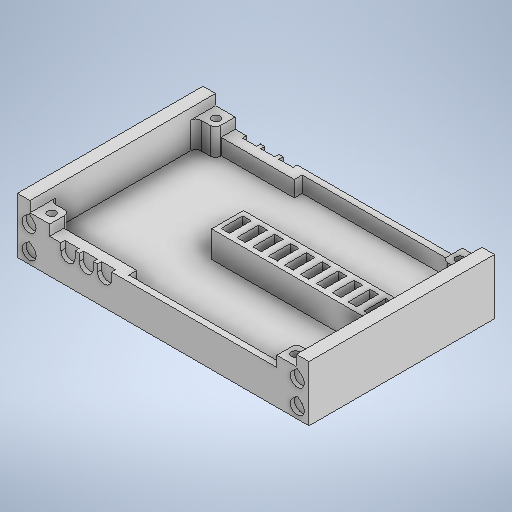
# Autodesk Inventor part: DisplayModuleHousing
Saved by Autodesk Inventor 2025.1 (Build 291241020, 241B)
## iProperties
Created: 2024-09-25
Part Number: DisplayModuleHousing
Material: Generic
Document SubType Name: Modeling
Designer: Si Teng Wu
Density: 1 g/cm^3
Appearance: Default
Author: Si Teng Wu
Autodesk Inventor part; units mm, degrees
ref_plane "YZ Plane" through (0, 0, 0) normal (1, 0, 0) x (0, 1, 0)
ref_plane "XZ Plane" through (0, 0, 0) normal (0, 1, 0) x (-1, 0, 0)
ref_plane "XY Plane" through (0, 0, 0) normal (0, 0, 1) x (1, 0, 0)
sketch "Sketch1" plane through (0, 0, 0) normal (0, 1, 0) x (-1, 0, 0)
  line L0 (55, 35) -> (-55, 35)
  line L1 (-55, 35) -> (-55, -35)
  line L2 (-55, -35) -> (55, -35)
  line L3 (55, -35) -> (55, 35)
  point P0 (0, 0)
  point P1 (-55, 0)
  point P2 (55, 0)
  dimension "d0" = 70
  dimension "d66" = 35
  dimension "d67" = 55
  dimension "d68" = 55
  constraints: 8 end point, 2 midpoint, 2 parallel, 1 horizontal, 1 perpendicular
  measures "d0" distance between parallel lines of L2 L0
  measures "d66" distance from line of L2 point (0, 0)
  measures "d67" distance of point (-55, 0) point (0, 0)
  measures "d68" distance of point (55, 0) point (0, 0)
extrude "Extrusion1" add sketch "Sketch1" along normal blind 21
sketch "Sketch2" plane through (0, 21, 0) normal (0, 1, 0) x (1, 0, 0)
  line L0 (-55, -35) -> (55, -35) projected
  line L1 (55, 35) -> (-55, 35) projected
  line L2 (50.25, -35) -> (-50.25, -35)
  line L3 (-50.25, -35) -> (-50.25, 35)
  line L4 (-50.25, 35) -> (50.25, 35)
  line L5 (50.25, 35) -> (50.25, -35)
  line L6 (-55, 35) -> (-55, -35) projected
  line L7 (55, -35) -> (55, 35) projected
  point P0 (0, 0)
  point P1 (-50.25, -35)
  dimension "d4" = 100.5
  dimension "d6" = 70
  dimension "d122" = 50.25
  constraints: 8 end point, 2 parallel, 2 point on line, 1 horizontal, 1 perpendicular
  measures "d4" distance between parallel lines of L3 L5
  measures "d6" distance between parallel lines of L1 L0
  measures "d122" distance from line of L3 point (0, 0)
extrude "Extrusion2" cut sketch "Sketch2" against normal blind 14 contours L3 L1 L5 L0
sketch "Sketch11" plane through (0, 7, 0) normal (0, 1, 0) x (1, 0, 0)
  line L0 (50.25, 35) -> (42.85, 35)
  line L1 (42.85, 35) -> (42.85, 27.5)
  line L2 (42.85, 27.5) -> (50.25, 27.5)
  line L3 (50.25, 27.5) -> (50.25, 35)
  circle A0 centre (46, 30.9) radius 1.55
  line L4 (50.25, 35) -> (50.25, -35) projected
  line L5 (50.25, -35) -> (42.85, -35)
  line L6 (42.85, -35) -> (42.85, -27.5)
  line L7 (42.85, -27.5) -> (50.25, -27.5)
  line L8 (50.25, -27.5) -> (50.25, -35)
  circle A1 centre (46, -31.1) radius 1.55
  line L9 (-42.85, 35) -> (-50.25, 35)
  line L10 (-50.25, 35) -> (-50.25, 27.5)
  line L11 (-50.25, 27.5) -> (-42.85, 27.5)
  line L12 (-42.85, 27.5) -> (-42.85, 35)
  circle A2 centre (-46, 30.9) radius 1.55
  line L13 (-50.25, 35) -> (50.25, 35) projected
  line L14 (-50.25, -35) -> (-50.25, 35) projected
  line L15 (-42.85, -35) -> (-50.25, -35)
  line L16 (-50.25, -35) -> (-50.25, -27.5)
  line L17 (-50.25, -27.5) -> (-42.85, -27.5)
  line L18 (-42.85, -27.5) -> (-42.85, -35)
  circle A3 centre (-46, -31.1) radius 1.55
  line L19 (50.25, -35) -> (-50.25, -35) projected
  point P0 (0, 0)
  point P1 (50.25, 31.25)
  point P2 (50.25, -8)
  point P3 (-42.85, 31.25)
  point P4 (-46.55, -35)
  point P5 (-50.25, -31.25)
  point P6 (50.25, -6)
  dimension "d89" = 7.5
  dimension "d91" = 3.1
  dimension "d92" = 4.25
  dimension "d93" = 7.4
  dimension "d334" = 3.9
  dimension "d335" = 7.5
  dimension "d336" = 7.4
  dimension "d338" = 92
  dimension "d339" = 62
  constraints: 32 end point, 8 parallel, 7 collinear, 4 centre point, 4 horizontal, 4 midpoint, 4 perpendicular, 3 equal radius, 2 horizontal alignment, 2 vertical alignment, 1 point on line
  measures "d89" distance between parallel lines of L17 L15
  measures "d91" diameter of A3
  measures "d92" distance from line of L16 A3.centre
  measures "d93" distance between parallel lines of L16 L18
  measures "d334" distance from line of L19 A3.centre
  measures "d335" distance between parallel lines of L11 L13
  measures "d336" distance between parallel lines of L6 L4
  measures "d338" distance of A0.centre A2.centre
  measures "d339" distance of A3.centre A2.centre
extrude "Extrusion10" add sketch "Sketch11" along normal blind 10 contours L3 L2 L1 L0 | L12 L11 L10 L9 | L4 L5 L6 L7 | L17 L18 L15 L14
fillet "Fillet5" radius 2 8 edges at (42.85, 12, 27.5) (50.25, 12, 27.5) (42.85, 12, -27.5) (50.25, 12, -27.5) (-42.85, 12, -27.5) (-50.25, 12, -27.5) (-50.25, 12, 27.5) (-42.85, 12, 27.5)
sketch "Sketch15" plane through (0, 7, 0) normal (0, 1, 0) x (1, 0, 0)
  circle A0 centre (46, -31.1) radius 1.55 projected
  circle A1 centre (46, -31.1) radius 1.6
  circle A2 centre (-46, -31.1) radius 1.55 projected
  circle A3 centre (-46, -31.1) radius 1.6
  circle A4 centre (-46, 30.9) radius 1.55 projected
  circle A5 centre (-46, 30.9) radius 1.6
  circle A6 centre (46, 30.9) radius 1.55 projected
  circle A7 centre (46, 30.9) radius 1.6
  point P0 (0, 0)
  constraints: 4 centre point, 4 coincident
extrude "Extrusion13" cut sketch "Sketch15" against normal through all contours A0 | A2 | A4 | A6
sketch "Sketch16" plane through (0, 0, 0) normal (0, -1, 0) x (1, 0, 0)
  line L0 (48.1, -28.2) -> (44.9, -28.2)
  line L1 (44.9, -28.2) -> (44.9, 28.2)
  line L2 (44.9, 28.2) -> (48.1, 28.2)
  line L3 (48.1, 28.2) -> (48.1, -28.2)
  line L4 (48.1, -28.2) -> (44.9, 28.2) construction
  line L5 (44.9, -28.2) -> (48.1, 28.2) construction
  line L6 (50.25, -25.5) -> (50.25, 25.5) projected
  line L7 (42.1, -28.2) -> (38.9, -28.2)
  line L8 (38.9, -28.2) -> (38.9, 28.2)
  line L9 (38.9, 28.2) -> (42.1, 28.2)
  line L10 (42.1, 28.2) -> (42.1, -28.2)
  line L11 (42.1, -28.2) -> (38.9, 28.2) construction
  line L12 (38.9, -28.2) -> (42.1, 28.2) construction
  line L13 (36.1, -28.2) -> (32.9, -28.2)
  line L14 (32.9, -28.2) -> (32.9, 28.2)
  line L15 (32.9, 28.2) -> (36.1, 28.2)
  line L16 (36.1, 28.2) -> (36.1, -28.2)
  line L17 (36.1, -28.2) -> (32.9, 28.2) construction
  line L18 (32.9, -28.2) -> (36.1, 28.2) construction
  line L19 (30.1, -28.2) -> (26.9, -28.2)
  line L20 (26.9, -28.2) -> (26.9, 28.2)
  line L21 (26.9, 28.2) -> (30.1, 28.2)
  line L22 (30.1, 28.2) -> (30.1, -28.2)
  line L23 (30.1, -28.2) -> (26.9, 28.2) construction
  line L24 (26.9, -28.2) -> (30.1, 28.2) construction
  line L25 (24.1, -28.2) -> (20.9, -28.2)
  line L26 (20.9, -28.2) -> (20.9, 28.2)
  line L27 (20.9, 28.2) -> (24.1, 28.2)
  line L28 (24.1, 28.2) -> (24.1, -28.2)
  line L29 (24.1, -28.2) -> (20.9, 28.2) construction
  line L30 (20.9, -28.2) -> (24.1, 28.2) construction
  line L31 (18.1, -28.2) -> (14.9, -28.2)
  line L32 (14.9, -28.2) -> (14.9, 28.2)
  line L33 (14.9, 28.2) -> (18.1, 28.2)
  line L34 (18.1, 28.2) -> (18.1, -28.2)
  line L35 (18.1, -28.2) -> (14.9, 28.2) construction
  line L36 (14.9, -28.2) -> (18.1, 28.2) construction
  line L37 (12.1, -28.2) -> (8.9, -28.2)
  line L38 (8.9, 28.2) -> (12.1, 28.2)
  line L39 (8.9, -28.2) -> (8.9, 28.2)
  line L40 (12.1, -28.2) -> (8.9, 28.2) construction
  line L41 (8.9, -28.2) -> (12.1, 28.2) construction
  line L42 (12.1, 28.2) -> (12.1, -28.2)
  line L43 (6.1, -28.2) -> (2.9, -28.2)
  line L44 (2.9, 28.2) -> (6.1, 28.2)
  line L45 (2.9, -28.2) -> (2.9, 28.2)
  line L46 (6.1, -28.2) -> (2.9, 28.2) construction
  line L47 (2.9, -28.2) -> (6.1, 28.2) construction
  line L48 (6.1, 28.2) -> (6.1, -28.2)
  line L49 (0.1, -28.2) -> (-3.1, -28.2)
  line L50 (-3.1, 28.2) -> (0.1, 28.2)
  line L51 (-3.1, -28.2) -> (-3.1, 28.2)
  line L52 (0.1, -28.2) -> (-3.1, 28.2) construction
  line L53 (-3.1, -28.2) -> (0.1, 28.2) construction
  line L54 (0.1, 28.2) -> (0.1, -28.2)
  line L55 (-5.9, -28.2) -> (-9.1, -28.2)
  line L56 (-9.1, 28.2) -> (-5.9, 28.2)
  line L57 (-9.1, -28.2) -> (-9.1, 28.2)
  line L58 (-5.9, -28.2) -> (-9.1, 28.2) construction
  line L59 (-9.1, -28.2) -> (-5.9, 28.2) construction
  line L60 (-5.9, 28.2) -> (-5.9, -28.2)
  line L61 (55, -35) -> (-55, -35) projected
  point P0 (46.5, 28.2)
  point P1 (40.5, 28.2)
  point P2 (34.5, 28.2)
  point P3 (28.5, 28.2)
  point P4 (22.5, 28.2)
  point P5 (16.5, 28.2)
  point P6 (10.5, 28.2)
  point P7 (4.5, 28.2)
  point P8 (-1.5, 28.2)
  point P9 (-7.5, 28.2)
  point P10 (46.5, -28.2)
  point P11 (40.5, 0)
  point P12 (46.5, 0)
  point P13 (34.5, 0)
  point P14 (40.5, 0)
  point P15 (28.5, 0)
  point P16 (34.5, 0)
  point P17 (22.5, 0)
  point P18 (28.5, 0)
  point P19 (16.5, 0)
  point P20 (22.5, 0)
  point P21 (10.5, 0)
  point P22 (16.5, 0)
  point P23 (4.5, 0)
  point P24 (10.5, 0)
  point P25 (-1.5, 0)
  point P26 (4.5, 0)
  point P27 (-7.5, 0)
  point P28 (-1.5, 0)
  point P29 (46.5, 0)
  dimension "d136" = 3.2
  dimension "d145" = 3.2
  dimension "d162" = 3.2
  dimension "d164" = 3.2
  dimension "d166" = 3.2
  dimension "d176" = 3.2
  dimension "d179" = 3.2
  dimension "d182" = 3.2
  dimension "d185" = 3.2
  dimension "d210" = 6
  dimension "d211" = 6
  dimension "d212" = 6
  dimension "d213" = 6
  dimension "d214" = 6
  dimension "d215" = 6
  dimension "d216" = 6
  dimension "d217" = 6
  dimension "d218" = 6
  dimension "d219" = 28.2
  dimension "d221" = 3.75
  dimension "d222" = 35
  constraints: 120 end point, 30 midpoint, 20 parallel, 19 collinear, 10 horizontal, 10 perpendicular
  measures "d136" distance between parallel lines of L1 L3
  measures "d145" distance between parallel lines of L14 L16
  measures "d162" distance between parallel lines of L20 L22
  measures "d164" distance between parallel lines of L26 L28
  measures "d166" distance between parallel lines of L32 L34
  measures "d176" distance between parallel lines of L39 L42
  measures "d179" distance between parallel lines of L45 L48
  measures "d182" distance between parallel lines of L51 L54
  measures "d185" distance between parallel lines of L57 L60
  measures "d210" distance of point (40.5, 0) point (46.5, 0)
  measures "d211" distance of point (34.5, 0) point (40.5, 0)
  measures "d212" distance of point (28.5, 0) point (34.5, 0)
  measures "d213" distance of point (22.5, 0) point (28.5, 0)
  measures "d214" distance of point (16.5, 0) point (22.5, 0)
  measures "d215" distance of point (10.5, 0) point (16.5, 0)
  measures "d216" distance of point (4.5, 0) point (10.5, 0)
  measures "d217" distance of point (-1.5, 0) point (4.5, 0)
  measures "d218" distance of point (-7.5, 0) point (-1.5, 0)
  measures "d219" distance from line of L0 point (46.5, 0)
  measures "d221" distance from line of L6 point (46.5, 0)
  measures "d222" distance from line of L61 point (46.5, 0)
extrude "Extrusion14" cut sketch "Sketch16" against normal blind 5
sketch "Sketch19" plane through (0, 7, 0) normal (0, 1, 0) x (1, 0, 0)
  line L0 (50.25, 35) -> (50.25, -35) projected
  line L1 (50.25, 6) -> (-10.75, 6)
  line L2 (-10.75, 6) -> (-10.75, -6)
  line L3 (-10.75, -6) -> (50.25, -6)
  line L4 (50.25, -6) -> (50.25, 6)
  line L5 (42.85, -35) -> (50.25, -35) projected
  point P0 (0, 0)
  dimension "d204" = 61
  dimension "d205" = 12
  dimension "d206" = 29
  constraints: 8 end point, 2 parallel, 1 horizontal, 1 perpendicular, 1 point on line
  measures "d204" distance between parallel lines of L2 L0
  measures "d205" distance between parallel lines of L3 L1
  measures "d206" distance between parallel lines of L5 L3
extrude "Extrusion16" add sketch "Sketch19" along normal up to surface (10 mm away)
sketch "Sketch17" plane through (0, 0, 0) normal (0, -1, 0) x (1, 0, 0)
  line L0 (48.1, 28.2) -> (48.1, -28.2) projected
  line L1 (44.9, 4.1) -> (48.1, 4.1)
  line L2 (48.1, 4.1) -> (48.1, -4.1)
  line L3 (48.1, -4.1) -> (44.9, -4.1)
  line L4 (44.9, -4.1) -> (44.9, 4.1)
  line L5 (44.9, 4.1) -> (48.1, -4.1) construction
  line L6 (48.1, 4.1) -> (44.9, -4.1) construction
  line L7 (44.9, -28.2) -> (44.9, 28.2) projected
  line L8 (42.1, 28.2) -> (42.1, -28.2) projected
  line L9 (38.9, 4.1) -> (42.1, 4.1)
  line L10 (42.1, 4.1) -> (42.1, -4.1)
  line L11 (42.1, -4.1) -> (38.9, -4.1)
  line L12 (38.9, -4.1) -> (38.9, 4.1)
  line L13 (38.9, 4.1) -> (42.1, -4.1) construction
  line L14 (42.1, 4.1) -> (38.9, -4.1) construction
  line L15 (36.1, 28.2) -> (36.1, -28.2) projected
  line L16 (32.9, 4.1) -> (36.1, 4.1)
  line L17 (36.1, 4.1) -> (36.1, -4.1)
  line L18 (36.1, -4.1) -> (32.9, -4.1)
  line L19 (32.9, -4.1) -> (32.9, 4.1)
  line L20 (32.9, 4.1) -> (36.1, -4.1) construction
  line L21 (36.1, 4.1) -> (32.9, -4.1) construction
  line L22 (30.1, 28.2) -> (30.1, -28.2) projected
  line L23 (26.9, 4.1) -> (30.1, 4.1)
  line L24 (30.1, 4.1) -> (30.1, -4.1)
  line L25 (30.1, -4.1) -> (26.9, -4.1)
  line L26 (26.9, -4.1) -> (26.9, 4.1)
  line L27 (26.9, 4.1) -> (30.1, -4.1) construction
  line L28 (30.1, 4.1) -> (26.9, -4.1) construction
  line L29 (24.1, 28.2) -> (24.1, -28.2) projected
  line L30 (20.9, 4.1) -> (24.1, 4.1)
  line L31 (24.1, 4.1) -> (24.1, -4.1)
  line L32 (24.1, -4.1) -> (20.9, -4.1)
  line L33 (20.9, -4.1) -> (20.9, 4.1)
  line L34 (20.9, 4.1) -> (24.1, -4.1) construction
  line L35 (24.1, 4.1) -> (20.9, -4.1) construction
  line L36 (18.1, 28.2) -> (18.1, -28.2) projected
  line L37 (14.9, 4.1) -> (18.1, 4.1)
  line L38 (18.1, 4.1) -> (18.1, -4.1)
  line L39 (18.1, -4.1) -> (14.9, -4.1)
  line L40 (14.9, -4.1) -> (14.9, 4.1)
  line L41 (14.9, 4.1) -> (18.1, -4.1) construction
  line L42 (18.1, 4.1) -> (14.9, -4.1) construction
  line L43 (12.1, 28.2) -> (12.1, -28.2) projected
  line L44 (8.9, 4.1) -> (12.1, 4.1)
  line L45 (12.1, 4.1) -> (12.1, -4.1)
  line L46 (12.1, -4.1) -> (8.9, -4.1)
  line L47 (8.9, -4.1) -> (8.9, 4.1)
  line L48 (8.9, 4.1) -> (12.1, -4.1) construction
  line L49 (12.1, 4.1) -> (8.9, -4.1) construction
  line L50 (2.9, 4.1) -> (6.1, 4.1)
  line L51 (6.1, 4.1) -> (6.1, -4.1)
  line L52 (6.1, -4.1) -> (2.9, -4.1)
  line L53 (2.9, -4.1) -> (2.9, 4.1)
  line L54 (2.9, 4.1) -> (6.1, -4.1) construction
  line L55 (6.1, 4.1) -> (2.9, -4.1) construction
  line L56 (-3.1, 4.1) -> (0.1, 4.1)
  line L57 (0.1, 4.1) -> (0.1, -4.1)
  line L58 (0.1, -4.1) -> (-3.1, -4.1)
  line L59 (-3.1, -4.1) -> (-3.1, 4.1)
  line L60 (-3.1, 4.1) -> (0.1, -4.1) construction
  line L61 (0.1, 4.1) -> (-3.1, -4.1) construction
  line L62 (-5.9, 28.2) -> (-5.9, -28.2) projected
  line L63 (-9.1, 4.1) -> (-5.9, 4.1)
  line L64 (-5.9, 4.1) -> (-5.9, -4.1)
  line L65 (-5.9, -4.1) -> (-9.1, -4.1)
  line L66 (-9.1, -4.1) -> (-9.1, 4.1)
  line L67 (-9.1, 4.1) -> (-5.9, -4.1) construction
  line L68 (-5.9, 4.1) -> (-9.1, -4.1) construction
  line L69 (38.9, -28.2) -> (38.9, 28.2) projected
  line L70 (32.9, -28.2) -> (32.9, 28.2) projected
  line L71 (26.9, -28.2) -> (26.9, 28.2) projected
  line L72 (20.9, -28.2) -> (20.9, 28.2) projected
  line L73 (14.9, -28.2) -> (14.9, 28.2) projected
  line L74 (8.9, -28.2) -> (8.9, 28.2) projected
  line L75 (2.9, -28.2) -> (2.9, 28.2) projected
  line L76 (-3.1, -28.2) -> (-3.1, 28.2) projected
  line L77 (0.1, 28.2) -> (0.1, -28.2) projected
  line L78 (6.1, 28.2) -> (6.1, -28.2) projected
  line L79 (12.1, 28.2) -> (12.1, -28.2) projected
  line L80 (-9.1, -28.2) -> (-9.1, 28.2) projected
  line L81 (55, -35) -> (-55, -35) projected
  point P0 (0, 0)
  point P1 (46.5, 0)
  point P2 (40.5, 0)
  point P3 (34.5, 0)
  point P4 (28.5, 0)
  point P5 (22.5, 0)
  point P6 (16.5, 0)
  point P7 (10.5, 0)
  point P8 (4.5, 0)
  point P9 (-1.5, 0)
  point P10 (-7.5, 0)
  point P11 (46.5, -4.1)
  point P12 (-5.9, 4.1)
  point P13 (12.1, 4.1)
  point P14 (24.1, 4.1)
  point P15 (42.1, 4.1)
  dimension "d200" = 4.1
  dimension "d201" = 35
  constraints: 120 end point, 23 collinear, 21 midpoint, 20 parallel, 16 point on line, 10 horizontal, 10 perpendicular
  measures "d200" distance of point (46.5, 0) point (46.5, -4.1)
  measures "d201" distance from line of L81 point (46.5, 0)
extrude "Extrusion15" cut sketch "Sketch17" against normal through all
chamfer "Chamfer3" distance 1 distance2 1.5 1 edges at (6.1, 5, -16.15) measured on face at (6.1, 1.6667, -20.1667)
chamfer "Chamfer4" distance 1 distance2 1.5 1 edges at (2.9, 5, -16.15) measured on face at (2.9, 1.6667, -12.1333)
chamfer "Chamfer5" distance 1 distance2 1.5 1 edges at (-3.1, 5, -16.15) measured on face at (-3.1, 1.6667, -12.1333)
chamfer "Chamfer6" distance 1 distance2 1.5 1 edges at (0.1, 5, -16.15) measured on face at (0.1, 1.6667, -20.1667)
chamfer "Chamfer7" distance 1 distance2 1.5 1 edges at (-5.9, 5, -16.15) measured on face at (-5.9, 1.6667, -20.1667)
chamfer "Chamfer8" distance 1 distance2 1.5 1 edges at (-9.1, 5, -16.15) measured on face at (-9.1, 1.6667, -12.1333)
chamfer "Chamfer9" distance 1 distance2 1.5 1 edges at (8.9, 5, -16.15) measured on face at (8.9, 1.6667, -12.1333)
chamfer "Chamfer10" distance 1 distance2 1.5 1 edges at (12.1, 5, -16.15) measured on face at (12.1, 1.6667, -20.1667)
chamfer "Chamfer11" distance 1 distance2 1.5 1 edges at (18.1, 5, -16.15) measured on face at (18.1, 1.6667, -20.1667)
chamfer "Chamfer12" distance 1 distance2 1.5 1 edges at (14.9, 5, -16.15) measured on face at (14.9, 3.3333, -20.1667)
chamfer "Chamfer13" distance 1 distance2 1.5 1 edges at (24.1, 5, -16.15) measured on face at (24.1, 1.6667, -20.1667)
chamfer "Chamfer14" distance 1 distance2 1.5 1 edges at (20.9, 5, -16.15) measured on face at (20.9, 1.6667, -12.1333)
chamfer "Chamfer15" distance 1 distance2 1.5 1 edges at (30.1, 5, -16.15) measured on face at (30.1, 1.6667, -20.1667)
chamfer "Chamfer16" distance 1 distance2 1.5 1 edges at (26.9, 5, -16.15) measured on face at (26.9, 1.6667, -12.1333)
chamfer "Chamfer17" distance 1 distance2 1.5 1 edges at (36.1, 5, -16.15) measured on face at (36.1, 1.6667, -20.1667)
chamfer "Chamfer18" distance 1 distance2 1.5 1 edges at (32.9, 5, -16.15) measured on face at (32.9, 1.6667, -12.1333)
chamfer "Chamfer19" distance 1 distance2 1.5 1 edges at (38.9, 5, -16.15) measured on face at (38.9, 1.6667, -12.1333)
chamfer "Chamfer20" distance 1 distance2 1.5 1 edges at (42.1, 5, -16.15) measured on face at (42.1, 1.6667, -20.1667)
chamfer "Chamfer21" distance 1.5 distance2 1 2 edges at (44.9, 5, -16.15) (48.1, 5, -16.15) measured on face at (45.9667, 5, -20.1667)
chamfer "Chamfer22" distance 1.5 distance2 1 2 edges at (44.9, 5, 16.15) (48.1, 5, 16.15) measured on face at (47.0333, 5, 12.1333)
chamfer "Chamfer23" distance 1.5 distance2 1 2 edges at (38.9, 5, 16.15) (42.1, 5, 16.15) measured on face at (39.9667, 5, 20.1667)
chamfer "Chamfer24" distance 1.5 distance2 1 2 edges at (32.9, 5, 16.15) (36.1, 5, 16.15) measured on face at (33.9667, 5, 20.1667)
chamfer "Chamfer25" distance 1.5 distance2 1 2 edges at (30.1, 5, 16.15) (26.9, 5, 16.15) measured on face at (27.9667, 5, 20.1667)
chamfer "Chamfer26" distance 1.5 distance2 1 2 edges at (20.9, 5, 16.15) (24.1, 5, 16.15) measured on face at (23.0333, 5, 12.1333)
chamfer "Chamfer27" distance 1.5 distance2 1 2 edges at (18.1, 5, 16.15) (14.9, 5, 16.15) measured on face at (15.9667, 5, 12.1333)
chamfer "Chamfer28" distance 1.5 distance2 1 2 edges at (8.9, 5, 16.15) (12.1, 5, 16.15) measured on face at (11.0333, 5, 12.1333)
chamfer "Chamfer29" distance 1.5 distance2 1 2 edges at (2.9, 5, 16.15) (6.1, 5, 16.15) measured on face at (5.0333, 5, 12.1333)
chamfer "Chamfer30" distance 1.5 distance2 1 2 edges at (-3.1, 5, 16.15) (0.1, 5, 16.15) measured on face at (-0.9667, 5, 12.1333)
chamfer "Chamfer31" distance 1.5 distance2 1 2 edges at (-5.9, 5, 16.15) (-9.1, 5, 16.15) measured on face at (-6.9667, 5, 12.1333)
sketch "Sketch20" plane through (0, 0, 0) normal (0, -1, 0) x (1, 0, 0)
  circle A0 centre (-46, -30.9) radius 1.55
  circle A1 centre (-46, -30.9) radius 1.55 projected
  circle A2 centre (-46, 31.1) radius 1.55
  circle A3 centre (46, 31.1) radius 1.55
  circle A4 centre (46, -30.9) radius 1.55
  circle A5 centre (-46, 31.1) radius 1.55 projected
  circle A6 centre (46, 31.1) radius 1.55 projected
  circle A7 centre (46, -30.9) radius 1.55 projected
  point P0 (0, 0)
  constraints: 4 centre point, 4 concentric, 4 equal radius
extrude "Extrusion17" add sketch "Sketch20" against normal blind 5
sketch "Sketch21" plane through (0, 7, 0) normal (0, 1, 0) x (1, 0, 0)
  line L0 (-42.85, -32.7) -> (42.85, -32.7)
  line L1 (42.85, -32.7) -> (42.85, -35)
  line L2 (42.85, -35) -> (-42.85, -35)
  line L3 (-42.85, -35) -> (-42.85, -32.7)
  line L4 (42.85, -35) -> (-42.85, -35) projected
  line L5 (-42.85, -35) -> (-42.85, -29.5) projected
  line L6 (42.85, -29.5) -> (42.85, -35) projected
  line L7 (-42.85, 35) -> (42.85, 35)
  line L8 (42.85, 35) -> (42.85, 32.7)
  line L9 (42.85, 32.7) -> (-42.85, 32.7)
  line L10 (-42.85, 32.7) -> (-42.85, 35)
  line L11 (-42.85, 29.5) -> (-42.85, 35) projected
  line L12 (-42.85, 35) -> (42.85, 35) projected
  line L13 (42.85, 35) -> (42.85, 29.5) projected
  line L14 (-42.85, -29.7) -> (-15.25, -29.7)
  line L15 (-15.25, -29.7) -> (-15.25, -32.7)
  line L16 (-15.25, -32.7) -> (-42.85, -32.7)
  line L17 (-42.85, -32.7) -> (-42.85, -29.7)
  line L18 (-42.85, 32.7) -> (-15.25, 32.7)
  line L19 (-15.25, 32.7) -> (-15.25, 29.7)
  line L20 (-15.25, 29.7) -> (-42.85, 29.7)
  line L21 (-42.85, 29.7) -> (-42.85, 32.7)
  line L22 (-50.25, -35) -> (-50.25, 35) projected
  point P0 (0, 0)
  point P1 (-15.25, 31.2)
  point P2 (-15.25, 32.7)
  dimension "d353" = 2.3
  dimension "d354" = 2.3
  dimension "d355" = 35
  dimension "d356" = 3
  dimension "d357" = 3
  constraints: 32 end point, 11 collinear, 8 parallel, 4 horizontal, 4 perpendicular, 1 midpoint
  measures "d353" distance between parallel lines of L0 L2
  measures "d354" distance between parallel lines of L9 L7
  measures "d355" distance from line of L22 point (-15.25, 31.2)
  measures "d356" distance between parallel lines of L18 L20
  measures "d357" distance between parallel lines of L0 L14
extrude "Extrusion18" add sketch "Sketch21" along normal blind 6
sketch "Sketch12" plane through (-42.85, 7, 35) normal (0, 0, 1) x (1, 0, 0)
  circle A0 centre (-7.75, 6) radius 2.65
  line L0 (-7.4, 10) -> (0, 10) projected
  line L1 (-12.15, -7) -> (-12.15, 14) projected
  circle A1 centre (93.45, 6) radius 2.65
  line L2 (97.85, -7) -> (97.85, 14) projected
  line L3 (85.7, 10) -> (93.1, 10) projected
  circle A2 centre (93.45, -3) radius 2.65
  circle A3 centre (-7.75, -3) radius 2.65
  line L4 (-9.4811, -0.9936) -> (-7.75, 0.5)
  line L5 (-7.75, 0.5) -> (-6.0189, -0.9936)
  line L6 (-9.4811, 8.0064) -> (-7.75, 9.5)
  line L7 (-7.75, 9.5) -> (-6.0189, 8.0064)
  line L8 (91.7189, -0.9936) -> (93.45, 0.5)
  line L9 (93.45, 0.5) -> (95.1811, -0.9936)
  line L10 (91.7189, 8.0064) -> (93.45, 9.5)
  line L11 (93.45, 9.5) -> (95.1811, 8.0064)
  line L12 (85.7, 0) -> (0, 0) projected
  line L13 (-12.15, -7) -> (97.85, -7) projected
  circle A4 centre (6.9, 3.35) radius 2.65
  circle A5 centre (13.8, 3.35) radius 2.65
  circle A6 centre (20.7, 3.35) radius 2.65
  line L14 (0, 6) -> (0, 0) projected
  line L15 (9.55, 3.35) -> (4.25, 3.35)
  line L16 (4.25, 3.35) -> (4.25, 6)
  line L17 (4.25, 6) -> (9.55, 6)
  line L18 (9.55, 6) -> (9.55, 3.35)
  line L19 (11.15, 3.35) -> (16.45, 3.35)
  line L20 (16.45, 3.35) -> (16.45, 6)
  line L21 (16.45, 6) -> (11.15, 6)
  line L22 (11.15, 6) -> (11.15, 3.35)
  line L23 (0, 6) -> (27.6, 6) projected
  line L24 (18.05, 3.35) -> (23.35, 3.35)
  line L25 (23.35, 3.35) -> (23.35, 6)
  line L26 (23.35, 6) -> (18.05, 6)
  line L27 (18.05, 6) -> (18.05, 3.35)
  line L28 (0, 6) -> (85.7, 6) projected
  point P0 (42.85, -7)
  point P1 (18.9615, 0)
  point P2 (22.4385, 0)
  point P3 (12.0615, 0)
  point P4 (15.5385, 0)
  point P5 (5.1615, 0)
  point P6 (8.6385, 0)
  point P7 (16.45, 3.35)
  point P8 (4.25, 3.35)
  point P9 (6.9, 3.35)
  point P10 (20.7, 6)
  point P11 (23.35, 3.35)
  point P12 (13.8, 6)
  point P13 (6.9, 6)
  point P14 (4.25, 3.35)
  dimension "d98" = 5.3
  dimension "d100" = 4
  dimension "d103" = 4.4
  dimension "d105" = 4.4
  dimension "d227" = 9
  dimension "d235" = 3.5
  dimension "d236" = 3.5
  dimension "d361" = 6.9
  dimension "d372" = 6.9
  dimension "d373" = 6.9
  dimension "d374" = 2.65
  constraints: 40 end point, 8 parallel, 8 point on circle, 8 tangent, 6 vertical alignment, 5 horizontal alignment, 4 centre point, 4 horizontal, 4 point on line, 4 vertical, 3 equal radius, 3 perpendicular, 1 midpoint, 11 other
  measures "d98" diameter of A0
  measures "d100" distance from line of L0 A0.centre
  measures "d103" distance from line of L1 A0.centre
  measures "d105" distance from line of L2 A1.centre
  measures "d227" distance of A0.centre A3.centre
  measures "d235" distance of A3.centre L4.end
  measures "d236" distance of A0.centre L6.end
  measures "d361" distance from line of L14 point (6.9, 3.35)
  measures "d372" distance of point (13.8, 3.35) point (6.9, 3.35)
  measures "d373" distance of point (20.7, 3.35) point (13.8, 3.35)
  measures "d374" distance from line of L23 point (6.9, 3.35)
extrude "Extrusion11" cut sketch "Sketch12" against normal blind 1.55
sketch "Sketch13" plane through (55, 0, -35) normal (0, 0, -1) x (-1, 0, 0)
  circle A0 centre (105.6, 13) radius 2.65
  circle A1 centre (4.4, 13) radius 2.65
  line L0 (97.85, 17) -> (105.25, 17) projected
  line L1 (110, 0) -> (110, 21) projected
  line L2 (4.75, 17) -> (12.15, 17) projected
  line L3 (0, 0) -> (0, 21) projected
  circle A2 centre (105.6, 4) radius 2.65
  circle A3 centre (4.4, 4) radius 2.65
  line L4 (6.1311, 15.0064) -> (4.4, 16.5)
  line L5 (4.4, 16.5) -> (2.6689, 15.0064)
  line L6 (6.1311, 6.0064) -> (4.4, 7.5)
  line L7 (4.4, 7.5) -> (2.6689, 6.0064)
  line L8 (103.8689, 6.0064) -> (105.6, 7.5)
  line L9 (105.6, 7.5) -> (107.3311, 6.0064)
  line L10 (103.8689, 15.0064) -> (105.6, 16.5)
  line L11 (105.6, 16.5) -> (107.3311, 15.0064)
  circle A4 centre (90.95, 10.35) radius 2.65
  circle A5 centre (84.05, 10.35) radius 2.65
  circle A6 centre (77.15, 10.35) radius 2.65
  line L12 (97.85, 13) -> (97.85, 17) projected
  line L13 (12.15, 13) -> (97.85, 13) projected
  line L14 (79.8, 10.35) -> (79.8, 13) projected
  line L15 (74.5, 10.35) -> (79.8, 10.35)
  line L16 (79.8, 10.35) -> (79.8, 13)
  line L17 (79.8, 13) -> (74.5, 13)
  line L18 (74.5, 13) -> (74.5, 10.35)
  line L19 (81.4, 10.35) -> (86.7, 10.35)
  line L20 (86.7, 10.35) -> (86.7, 13)
  line L21 (86.7, 13) -> (81.4, 13)
  line L22 (81.4, 13) -> (81.4, 10.35)
  line L23 (93.6, 10.35) -> (93.6, 13) projected
  line L24 (88.3, 10.35) -> (93.6, 10.35)
  line L25 (93.6, 10.35) -> (93.6, 13)
  line L26 (93.6, 13) -> (88.3, 13)
  line L27 (88.3, 13) -> (88.3, 10.35)
  point P0 (55, 0)
  point P1 (90.95, 13)
  point P2 (84.05, 13)
  point P3 (77.15, 13)
  dimension "d109" = 4.4
  dimension "d110" = 5.3
  dimension "d111" = 4
  dimension "d233" = 4.4
  dimension "d234" = 9
  dimension "d241" = 3.5
  dimension "d365" = 3.5
  dimension "d375" = 6.9
  dimension "d376" = 6.9
  dimension "d377" = 6.9
  dimension "d378" = 2.65
  constraints: 40 end point, 10 parallel, 10 point on circle, 9 tangent, 6 centre point, 6 vertical alignment, 5 horizontal alignment, 3 equal radius, 3 horizontal, 3 perpendicular, 3 point on line, 1 vertical, 5 other
  measures "d109" distance from line of L1 A0.centre
  measures "d110" diameter of A1
  measures "d111" distance from line of L2 A1.centre
  measures "d233" distance from line of L3 A3.centre
  measures "d234" distance of A3.centre A1.centre
  measures "d241" distance of A1.centre L4.end
  measures "d365" distance of L6.end A3.centre
  measures "d375" distance from line of L12 A4.centre
  measures "d376" distance of point (84.05, 10.35) A4.centre
  measures "d377" distance of A6.centre point (84.05, 10.35)
  measures "d378" distance from line of L13 A4.centre
extrude "Extrusion12" cut sketch "Sketch13" against normal blind 1.55
body "Solid1"
